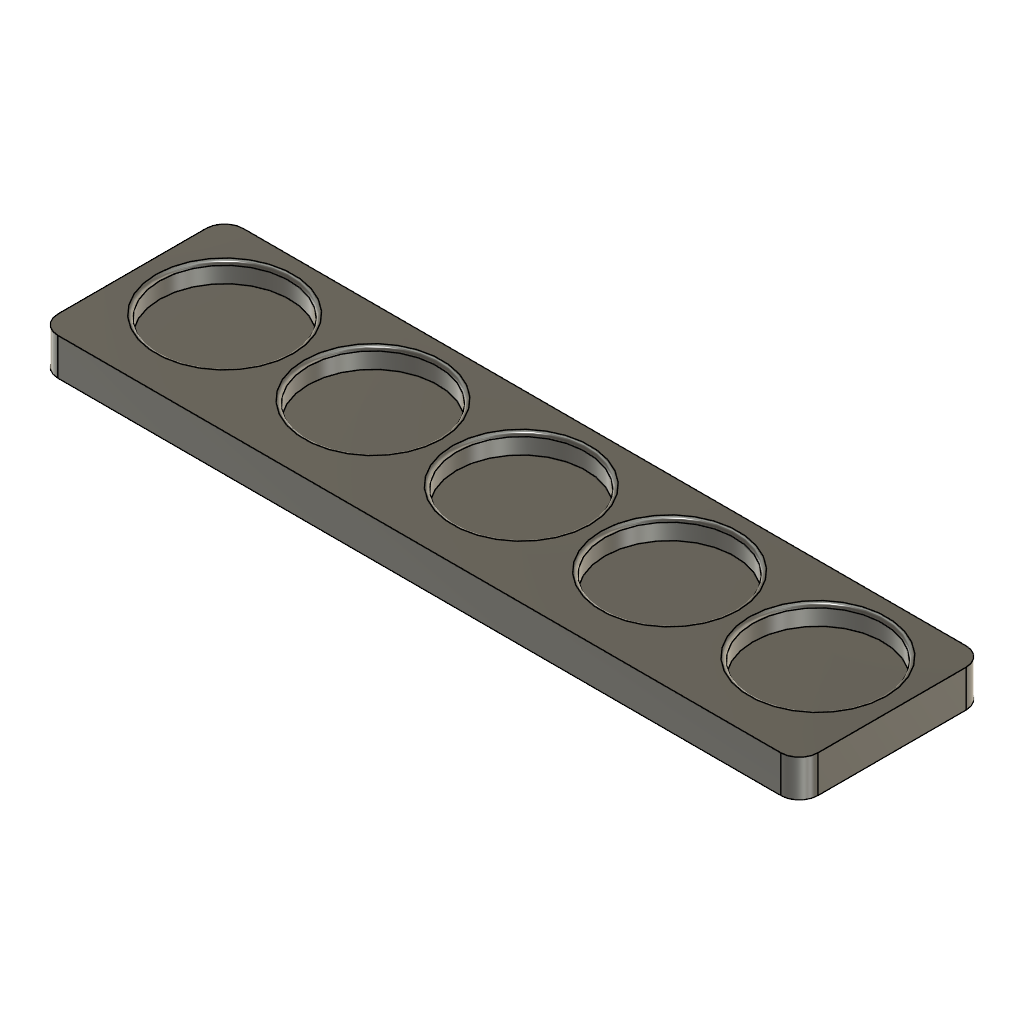
coin-capsule-holder (Autodesk Fusion 360 design; units mm, degrees)
part number: 2025-11-09-20-00-10-040
Autodesk Fusion 360 part; units mm, degrees
sketch "Sketch1" plane through (0, 0, 0) normal (0, 0, 1) x (1, 0, 0)
  line L0 (0, 0) -> (235, 0)
  line L1 (235, 0) -> (235, 55)
  line L2 (235, 55) -> (0, 55)
  line L3 (0, 55) -> (0, 0)
  circle A0 centre (27.5, 32.5) radius 17.5
  circle A1 centre (67.5, 32.5) radius 17.5
  circle A2 centre (107.5, 32.5) radius 17.5
  circle A3 centre (147.5, 32.5) radius 17.5
  circle A4 centre (187.5, 32.5) radius 17.5
  dimension "d1" = 235
  dimension "d2" = 55
  dimension "d9" = 35
  dimension "d10" = 35
  dimension "d11" = 35
  dimension "d12" = 35
  dimension "d13" = 35
  constraint horizontal L0
  constraint vertical L1
  constraint horizontal L2
  constraint vertical L3
  constraint coincident L0.start L3.end
  measures "d1" distance of L0.start L0.end
  measures "d2" distance of L0.start L2.end
  measures "d9" diameter of A0
  measures "d10" diameter of A1
  measures "d11" diameter of A2
  measures "d12" diameter of A3
  measures "d13" diameter of A4
extrude "Extrude1" add sketch "Sketch1" along normal blind 10
extrude "Extrude2" add sketch "Sketch1" along normal blind 4.7 contours A0 | A1 | A2 | A3 | A4
extrude "Extrude3" cut 1 faces at (235, 18.3333, 3.3333) along direction (-1, 0, 0) blind 20
extrude "Extrude4" cut 1 faces at (215, 18.3333, 3.3333) along direction (-1, 0, 0) blind 5
extrude "Extrude5" cut 1 faces at (0, 36.6667, 3.3333) along direction (1, 0, 0) blind 5
extrude "Extrude6" cut 1 faces at (73.3333, 0, 3.3333) along direction (0, 1, 0) blind 5
fillet "Fillet3" radius 1 5 edges at (11.1843, 38.8283, 10) (51.1843, 38.8283, 10) (91.1843, 38.8283, 10) (131.1843, 38.8283, 10) (171.1843, 38.8283, 10)
fillet "Fillet4" radius 5 4 edges at (210, 5, 5) (5, 5, 5) (5, 55, 5) (210, 55, 5)
